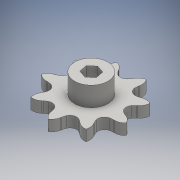
# Autodesk Inventor part: sprocket9teeth
Saved by Autodesk Inventor 2016 (Build 200138000, 138)
## iProperties
Created: 2016-10-17
Part Number: sprocket9teeth
Material: Generic
Document SubType Name: Modeling
Designer: Kevin G
Density: 1 g/cm^3
Appearance: Default
Author: Kevin G
Autodesk Inventor part; units mm, degrees
ref_plane "YZ Plane" through (0, 0, 0) normal (1, 0, 0) x (0, 1, 0)
ref_plane "XZ Plane" through (0, 0, 0) normal (0, 1, 0) x (-1, 0, 0)
ref_plane "XY Plane" through (0, 0, 0) normal (0, 0, 1) x (1, 0, 0)
sketch "Sketch1" plane through (0, 0, 0) normal (0, 0, 1) x (1, 0, 0)
  circle A0 centre (-7.6113, 0) radius 13.9246
  line L0 (-7.6113, 0) -> (-7.6113, 20.3737) construction
  line L1 (-31.3316, 0) -> (16.109, 0) projected
  arc A1 (-10.3449, 13.3103) -> (-9.5382, 12.2099) centre (-4.6027, 16.6739) ccw
  line L2 (-10.3449, 13.3103) -> (-10.5401, 13.65)
  arc A2 (-9.5382, 12.2099) -> (-7.6113, 11.3452) centre (-7.6113, 13.9246) ccw
  arc A3 (-10.5214, 13.6171) -> (-13.3307, 15.7138) centre (-14.2944, 11.4922) ccw
  arc A4 (-5.6845, 12.2099) -> (-4.8778, 13.3103) centre (-10.6199, 16.6739) ccw
  line L3 (-4.8778, 13.3103) -> (-4.6825, 13.65)
  arc A5 (-7.6113, 11.3452) -> (-5.6845, 12.2099) centre (-7.6113, 13.9246) ccw
  arc A6 (-1.892, 15.7138) -> (-4.7012, 13.6171) centre (-0.9282, 11.4922) ccw
  arc A7 (-18.5935, 8.5607) -> (-22.0932, 8.3611) centre (-20.1179, 4.5077) ccw
  arc A8 (-18.261, 8.4392) -> (-16.9357, 8.1147) centre (-16.0244, 14.7068) ccw
  line L4 (-18.261, 8.4392) -> (-18.629, 8.5739)
  arc A9 (-16.9357, 8.1147) -> (-14.9039, 8.691) centre (-16.5619, 10.6669) ccw
  arc A10 (-14.9039, 8.691) -> (-13.9836, 10.5919) centre (-16.5619, 10.6669) ccw
  arc A11 (-13.9836, 10.5919) -> (-14.073, 11.9533) centre (-20.6338, 10.8391) ccw
  line L5 (-14.073, 11.9533) -> (-14.1417, 12.3391)
  arc A12 (-13.3307, 15.7138) -> (-14.1349, 12.3019) centre (-9.8788, 13.0993) ccw
  arc A13 (-21.5269, -0.5013) -> (-24.0795, -2.9038) centre (-20.0894, -4.586) ccw
  arc A14 (-21.194, -0.3807) -> (-19.9703, 0.2226) centre (-23.5095, 5.8583) ccw
  line L6 (-21.194, -0.3807) -> (-21.5625, -0.514)
  arc A15 (-19.9703, 0.2226) -> (-18.7842, 1.9701) centre (-21.3244, 2.418) ccw
  arc A16 (-18.7842, 1.9701) -> (-19.3011, 4.0178) centre (-21.3244, 2.418) ccw
  arc A17 (-19.3011, 4.0178) -> (-20.2447, 5.0033) centre (-24.5544, -0.0675) ccw
  line L7 (-20.2447, 5.0033) -> (-20.5454, 5.2546)
  arc A18 (-22.0932, 8.3611) -> (-20.5162, 5.2305) centre (-17.7684, 8.5772) ccw
  arc A19 (-17.949, -9.3288) -> (-18.3602, -12.81) centre (-14.2223, -11.5338) ccw
  arc A20 (-17.7716, -9.0224) -> (-17.2219, -7.7736) centre (-23.5556, -5.7315) ccw
  line L8 (-17.7716, -9.0224) -> (-17.9681, -9.3614)
  arc A21 (-17.2219, -7.7736) -> (-17.4366, -5.6726) centre (-19.6704, -6.9623) ccw
  arc A22 (-17.4366, -5.6726) -> (-19.1488, -4.4362) centre (-19.6704, -6.9623) ccw
  arc A23 (-19.1488, -4.4362) -> (-20.5051, -4.2878) centre (-20.5471, -10.9425) ccw
  line L9 (-20.5051, -4.2878) -> (-20.897, -4.2886)
  arc A24 (-24.0795, -2.9038) -> (-20.8592, -4.2883) centre (-20.9054, 0.0416) ccw
  arc A25 (-9.534, -13.7912) -> (-7.6113, -16.7222) centre (-5.2618, -13.0849) ccw
  arc A26 (-9.595, -13.4425) -> (-9.9767, -12.1325) centre (-16.1413, -14.6394) ccw
  line L10 (-9.595, -13.4425) -> (-9.5277, -13.8285)
  arc A27 (-9.9767, -12.1325) -> (-11.4916, -10.661) centre (-12.3738, -13.0849) ccw
  arc A28 (-11.4916, -10.661) -> (-13.598, -10.8145) centre (-12.3738, -13.0849) ccw
  arc A29 (-13.598, -10.8145) -> (-14.7324, -11.5726) centre (-10.487, -16.6974) ccw
  line L11 (-14.7324, -11.5726) -> (-15.0321, -11.8251)
  arc A30 (-18.3602, -12.81) -> (-15.0033, -11.8006) centre (-17.8219, -8.5134) ccw
  arc A31 (-0.2194, -11.8006) -> (3.1375, -12.81) centre (2.5993, -8.5134) ccw
  arc A32 (-0.4902, -11.5726) -> (-1.6246, -10.8145) centre (-4.7356, -16.6974) ccw
  line L12 (-0.4902, -11.5726) -> (-0.1905, -11.8251)
  arc A33 (-1.6246, -10.8145) -> (-3.731, -10.661) centre (-2.8488, -13.0849) ccw
  arc A34 (-3.731, -10.661) -> (-5.2459, -12.1325) centre (-2.8488, -13.0849) ccw
  arc A35 (-5.2459, -12.1325) -> (-5.6276, -13.4425) centre (0.9186, -14.6394) ccw
  line L13 (-5.6276, -13.4425) -> (-5.6949, -13.8285)
  arc A36 (-7.6113, -16.7222) -> (-5.6886, -13.7912) centre (-9.9608, -13.0849) ccw
  arc A37 (5.6365, -4.2883) -> (8.8569, -2.9038) centre (5.6827, 0.0416) ccw
  arc A38 (5.2825, -4.2878) -> (3.9262, -4.4362) centre (5.3244, -10.9425) ccw
  line L14 (5.2825, -4.2878) -> (5.6744, -4.2886)
  arc A39 (3.9262, -4.4362) -> (2.214, -5.6726) centre (4.4478, -6.9623) ccw
  arc A40 (2.214, -5.6726) -> (1.9993, -7.7736) centre (4.4478, -6.9623) ccw
  arc A41 (1.9993, -7.7736) -> (2.5489, -9.0224) centre (8.333, -5.7315) ccw
  line L15 (2.5489, -9.0224) -> (2.7455, -9.3614)
  arc A42 (3.1375, -12.81) -> (2.7264, -9.3288) centre (-1.0003, -11.5338) ccw
  arc A43 (5.2936, 5.2305) -> (6.8706, 8.3611) centre (2.5458, 8.5772) ccw
  arc A44 (5.0221, 5.0033) -> (4.0785, 4.0178) centre (9.3317, -0.0675) ccw
  line L16 (5.0221, 5.0033) -> (5.3227, 5.2546)
  arc A45 (4.0785, 4.0178) -> (3.5616, 1.9701) centre (6.1018, 2.418) ccw
  arc A46 (3.5616, 1.9701) -> (4.7477, 0.2226) centre (6.1018, 2.418) ccw
  arc A47 (4.7477, 0.2226) -> (5.9714, -0.3807) centre (8.2869, 5.8583) ccw
  line L17 (5.9714, -0.3807) -> (6.3399, -0.514)
  arc A48 (8.8569, -2.9038) -> (6.3043, -0.5013) centre (4.8668, -4.586) ccw
  arc A49 (-1.0877, 12.3019) -> (-1.892, 15.7138) centre (-5.3438, 13.0993) ccw
  arc A50 (-1.1497, 11.9533) -> (-1.239, 10.5919) centre (5.4112, 10.8391) ccw
  line L18 (-1.1497, 11.9533) -> (-1.0809, 12.3391)
  arc A51 (-1.239, 10.5919) -> (-0.3187, 8.691) centre (1.3393, 10.6669) ccw
  arc A52 (-0.3187, 8.691) -> (1.7131, 8.1147) centre (1.3393, 10.6669) ccw
  arc A53 (1.7131, 8.1147) -> (3.0384, 8.4392) centre (0.8018, 14.7068) ccw
  line L19 (3.0384, 8.4392) -> (3.4064, 8.5739)
  arc A54 (6.8706, 8.3611) -> (3.3709, 8.5607) centre (4.8953, 4.5077) ccw
  point P0 (0, 0)
  dimension "d0" = 27.8492
  constraints: 128 point on circle, 55 centre point, 38 end point, 7 symmetric about line, 2 point on line, 1 tangent, 1 vertical, 3 other
  measures "d0" diameter of A0
extrude "Extrusion1" add sketch "Sketch1" along normal blind 4.2767 contours L16 A44 A45 A46 A47 L1 A14 A15 A16 A17 L7 A0 L4 A8 A9 A10 A11 L5 L2 A1 A2 A5 A4 L3 L18 A50 A51 A52 A53 L19 | A0 L19 A54 A43 | L17 A48 A37 A0 | A0 L14 A38 A39 A40 A41 L15 L12 A32 A33 A34 A35 L13 L10 A26 A27 A28 A29 L11 L8 A20 A21 A22 A23 L9 L6 A14 L1 A47 L17 | A0 L3 A6 A49 | L15 A42 A31 A0 | L7 A18 A7 A0 | A0 L9 A24 A13 | A0 L5 A12 A3 L2 | L13 A36 A25 A0 | A0 L11 A30 A19
sketch "Sketch2" plane through (0, 0, 4.2767) normal (0, 0, 1) x (1, 0, 0)
  circle A0 centre (-7.6113, 0) radius 6.4665
  point P0 (0, 0)
  constraints: 1 centre point
extrude "Extrusion2" add sketch "Sketch2" along normal blind 7.62
sketch "Sketch3" plane through (-7.6113, 0, 11.8967) normal (0, 0, 1) x (1, 0, 0)
  line L0 (-3, 1) -> (-0.634, 3.0981)
  line L1 (-0.634, 3.0981) -> (2.366, 2.0981)
  line L2 (2.366, 2.0981) -> (3, -1)
  line L3 (3, -1) -> (0.634, -3.0981)
  line L4 (0.634, -3.0981) -> (-2.366, -2.0981)
  line L5 (-2.366, -2.0981) -> (-3, 1)
  point P0 (7.6113, 0)
  point P1 (0, 0)
  constraints: 12 end point, 13 other
emboss "Emboss1" sketch "Sketch3" operation cut depth 12.62 direction (0, 0, -1)
body "Solid1"
